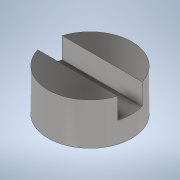
# Autodesk Inventor part: screw
Saved by Autodesk Inventor 2021 (Build 250183000, 183)
## iProperties
Created: 2021-07-07
Part Number: screw
Material: Steel, High Strength, Low Alloy
Document SubType Name: Modeling
Designer: VK
Density: 7.85 g/cm^3
Appearance: Steel - Polished
Author: VK
Autodesk Inventor part; units mm, degrees
ref_plane "YZ Plane" through (0, 0, 0) normal (1, 0, 0) x (0, 1, 0)
ref_plane "XZ Plane" through (0, 0, 0) normal (0, 1, 0) x (-1, 0, 0)
ref_plane "XY Plane" through (0, 0, 0) normal (0, 0, 1) x (1, 0, 0)
sketch "Sketch1" plane through (0, 0, 0) normal (0, 1, 0) x (-1, 0, 0)
  circle A0 centre (0, 0) radius 1
  dimension "d0" = 2
  constraints: 1 centre point, 1 coincident
  measures "d0" diameter of A0
extrude "Extrusion1" add sketch "Sketch1" along normal blind 1
sketch "Sketch2" plane through (0, 1, 0) normal (0, 1, 0) x (1, 0, 0)
  line L0 (-1, -0.2916) -> (1, -0.2916)
  line L1 (1, -0.2916) -> (1, 0.2916)
  line L2 (1, 0.2916) -> (-1, 0.2916)
  line L3 (-1, 0.2916) -> (-1, -0.2916)
  line L4 (-1, -0.2916) -> (1, 0.2916) construction
  line L5 (1, -0.2916) -> (-1, 0.2916) construction
  point P0 (0, 0)
  constraints: 12 end point, 2 midpoint, 2 parallel, 1 horizontal, 1 perpendicular
extrude "Extrusion2" cut sketch "Sketch2" against normal blind 0.5
body "Solid1"
